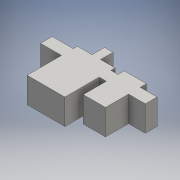
# Autodesk Inventor part: FR_bounding_box
Saved by Autodesk Inventor 2016 (Build 200138000, 138)
## iProperties
Created: 2016-10-18
Part Number: FR_bounding_box
Material: Generic
Document SubType Name: Modeling
Designer: rawrdong
Density: 1 g/cm^3
Appearance: Default
Author: rawrdong
Autodesk Inventor part; units mm, degrees
ref_plane "YZ Plane" through (0, 0, 0) normal (1, 0, 0) x (0, 1, 0)
ref_plane "XZ Plane" through (0, 0, 0) normal (0, 1, 0) x (-1, 0, 0)
ref_plane "XY Plane" through (0, 0, 0) normal (0, 0, 1) x (1, 0, 0)
sketch "Sketch1" plane through (0, 0, 0) normal (0, 0, 1) x (1, 0, 0)
  line L0 (0, 0) -> (50, 0)
  line L1 (50, 0) -> (50, 10)
  line L2 (50, 10) -> (140, 10)
  line L3 (140, 10) -> (140, 0)
  line L4 (140, 0) -> (157, 0)
  line L5 (157, 0) -> (157, 15)
  line L6 (157, 15) -> (210, 15)
  line L7 (210, 15) -> (210, 0)
  line L8 (210, 0) -> (250, 0)
  line L9 (250, 0) -> (250, -28)
  line L10 (250, -28) -> (210, -28)
  line L11 (210, -28) -> (210, -83)
  line L12 (210, -83) -> (157, -83)
  line L13 (157, -83) -> (157, -28)
  line L14 (157, -28) -> (140, -28)
  line L15 (140, -28) -> (140, -110)
  line L16 (140, -110) -> (50, -110)
  line L17 (50, -110) -> (50, -28)
  line L18 (50, -28) -> (0, -28)
  line L19 (0, -28) -> (0, 0)
  line L20 (85, 10) -> (105, 10)
  line L21 (105, 10) -> (105, 40)
  line L22 (105, 40) -> (85, 40)
  line L23 (85, 40) -> (85, 10)
  point P0 (95, 10)
  point P1 (95, 40)
  dimension "d0" = 90
  dimension "d1" = 53
  dimension "d2" = 17
  dimension "d3" = 40
  dimension "d4" = 50
  dimension "d5" = 10
  dimension "d6" = 15
  dimension "d9" = 28
  dimension "d10" = 110
  dimension "d11" = 83
  dimension "d14" = 30
  dimension "d15" = 20
  constraints: 48 end point, 14 point on line, 12 perpendicular, 3 parallel, 2 horizontal, 2 midpoint, 2 vertical alignment, 1 collinear, 1 vertical
  measures "d0" distance of L1.end L2.end
  measures "d1" distance of L5.end L6.end
  measures "d2" distance of L3.end L4.end
  measures "d3" distance of L7.end L8.end
  measures "d4" distance of L0.start L0.end
  measures "d5" distance of L0.end L1.end
  measures "d6" distance between parallel lines of L0 L6
  measures "d9" distance of L18.end L0.start
  measures "d10" distance between parallel lines of L0 L16
  measures "d11" distance between parallel lines of L8 L12
  measures "d14" distance of L20.end L21.end
  measures "d15" distance of L21.end L22.end
extrude "Extrusion1" add sketch "Sketch1" along normal blind 61
body "Solid1"
